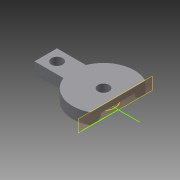
# Autodesk Inventor part: tiedown-hook-mount-clip
Saved by Autodesk Inventor 2015 (Build 190159000, 159)
## iProperties
Created: 2015-02-01
Part Number: tiedown-hook-mount-clip
Material: Generic
Document SubType Name: Modeling
Designer: bovine
Density: 1 g/cm^3
Appearance: Default
Author: bovine
Autodesk Inventor part; units mm, degrees
ref_plane "YZ Plane" through (0, 0, 0) normal (1, 0, 0) x (0, 1, 0)
ref_plane "XZ Plane" through (0, 0, 0) normal (0, 1, 0) x (-1, 0, 0)
ref_plane "XY Plane" through (0, 0, 0) normal (0, 0, 1) x (1, 0, 0)
sketch "SketchCircles" plane through (0, 0, 0) normal (0, 1, 0) x (-1, 0, 0)
  circle A0 centre (0, 0) radius 12.7
  circle A1 centre (0, 0) radius 6.35
  line L0 (32.5969, -6.35) -> (16.267, -6.35)
  line L1 (16.267, 6.35) -> (32.5969, 6.35)
  line L2 (32.5969, 6.35) -> (32.5969, -6.35)
  line L3 (32.5969, -6.35) -> (15.4107, 6.35) construction
  line L4 (15.4107, -6.35) -> (32.5969, 6.35) construction
  arc A2 (16.267, 6.35) -> (16.267, -6.35) centre (0, 0) ccw
  point P0 (24.0038, 0)
  dimension "d0" = 25.4
  dimension "d1" = 12.7
  constraints: 10 end point, 3 centre point, 3 coincident, 2 midpoint, 2 point on circle, 1 horizontal, 1 parallel
  measures "d0" diameter of A0
  measures "d1" diameter of A1
extrude "Extrusion100" add sketch "SketchCircles" along normal blind 6.35 contours A0 | A1 | L0 A2 L1 L2
sketch "SketchLines" plane through (0, 0, 0) normal (0, -1, 0) x (1, 0, 0)
  line L0 (-17.7365, 0) -> (17.5532, 0)
  line L1 (-0.0917, 17.7823) -> (-0.0917, -17.324)
  point P0 (0, 0)
  constraints: 4 end point, 1 horizontal, 1 vertical
hole "Hole1" at (0, 0, 0) direction (0, 1, 0) diameter 25.4 depth 3.175
sketch "Sketch3" plane through (0, 3.175, 0) normal (0, -1, 0) x (1, 0, 0)
  circle A0 centre (0, 0) radius 6.35
  dimension "d12" = 12.7
  constraints: 1 centre point, 1 coincident
  measures "d12" diameter of A0
extrude "Extrusion2" add sketch "Sketch3" along normal blind 3.175
chamfer "Chamfer1" distance 1.397 angle 45 1 edges at (0, 0, 12.7)
chamfer "Chamfer2" distance 1.397 angle 45 1 edges at (-6.35, 0, 0)
sketch "Sketch4" plane through (0, 6.35, 0) normal (0, 1, 0) x (1, 0, 0)
  circle A0 centre (0, 0) radius 3.9688
  point P0 (0, 0)
  dimension "d21" = 7.9375
  constraints: 1 centre point, 1 coincident
  measures "d21" diameter of A0
hole "Hole2" at (0, 6.35, 0) direction (0, -1, 0) diameter 6.35 depth 12.7
sketch "Sketch5" plane through (0, 0, 0) normal (0, -1, 0) x (1, 0, 0)
  line L0 (-18.8474, 0) -> (20.3869, 0)
  circle A0 centre (0, 0) radius 6.35 projected
  line L1 (-18.8474, 0) -> (-26.1971, 0)
  line L2 (8.1484, 0) -> (8.1484, 20.5164)
  point P0 (0, 0)
  point P1 (6.35, 0)
  constraints: 6 end point, 2 horizontal, 2 point on line, 1 horizontal alignment, 1 perpendicular, 1 other
hole "Hole3" at (-26.1971, 0, 0) direction (0, 1, 0) diameter 6.35 end through all
ref_plane "Work Plane4" through (8.1484, 0, 0) normal (1, 0, 0) x (0, 0, 1)
split "Split2" plane through (8.1484, 0, 0) removes the side toward (1, 0, 0)
body "Solid1"
